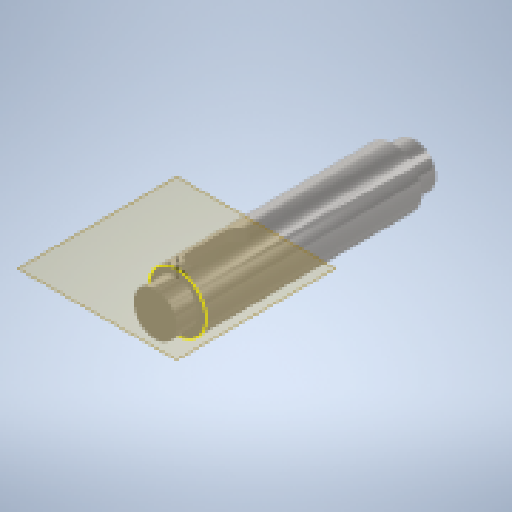
# Autodesk Inventor part: 入力軸
Saved by Autodesk Inventor 2024 (Build 280153000, 153)
## iProperties
Created: 2023-05-29
Part Number: 入力軸
Material: 鋼、炭素鋼
Document SubType Name: Modeling
Designer: yuta2
Density: 7.85 g/cm^3
Appearance: 半つや出し
Mass: 16.8186 g
Surface Area: 12.4913 cm^2
Volume: 2.1425 cm^3
Author: yuta2
Autodesk Inventor part; units mm, degrees
ref_plane "YZ Plane" through (0, 0, 0) normal (1, 0, 0) x (0, 1, 0)
ref_plane "XZ Plane" through (0, 0, 0) normal (0, 1, 0) x (-1, 0, 0)
ref_plane "XY Plane" through (0, 0, 0) normal (0, 0, 1) x (1, 0, 0)
sketch "スケッチ1" plane through (0, 0, 0) normal (1, 0, 0) x (0, 1, 0)
  line L0 (0, 0) -> (3, 0)
  line L1 (3, 0) -> (3, 3)
  line L2 (3, 3) -> (0, 3)
  line L3 (0, 3) -> (0, 0)
  line L4 (0, 0) -> (4, 0)
  line L5 (4, 0) -> (4, -37)
  line L6 (4, -37) -> (0, -37)
  line L7 (0, -37) -> (0, 0)
  line L8 (0, -37) -> (3, -37)
  line L9 (3, -37) -> (3, -40)
  line L10 (3, -40) -> (0, -40)
  line L11 (0, -40) -> (0, -37)
  dimension "d0" = 3
  dimension "d1" = 3
  dimension "d2" = 4
  dimension "d3" = 37
  dimension "d4" = 3
  dimension "d5" = 3
  constraints: 24 end point, 6 parallel, 3 horizontal, 3 perpendicular
  measures "d0" distance of L2.end L1.end
  measures "d1" distance of L1.end L0.end
  measures "d2" distance of L5.end L6.end
  measures "d3" distance of L4.end L5.end
  measures "d4" distance of L9.end L10.end
  measures "d5" distance of L8.end L9.end
revolve "回転1" add sketch "スケッチ1" angle 360 about axis through (0, 0, -37) along (0, 0, 1)
sketch "スケッチ2" plane through (0, 0, 0) normal (0, 0, 1) x (1, 0, 0)
  circle A0 centre (0, 0) radius 4 projected
  point P0 (0, 4)
  constraints: 2 vertical alignment, 1 other
ref_plane "作業平面1" through (0, 4, 0) normal (0, 1, 0) x (-1, 0, 0)
sketch "スケッチ3" plane through (0, 4, 0) normal (0, 1, 0) x (-1, 0, 0)
  line L0 (0, 0) -> (0, 3)
  line L1 (3, 3) -> (-3, 3) projected
  line L2 (1.5, -3) -> (-1.5, -3)
  line L3 (-1.5, -3) -> (-1.5, -8)
  line L4 (-1.5, -8) -> (1.5, -8)
  line L5 (1.5, -8) -> (1.5, -3)
  line L6 (4, 0) -> (-4, 0) projected
  circle A0 centre (0, -3) radius 1.5
  circle A1 centre (0, -8) radius 1.5
  line L7 (-1.5, -27) -> (1.5, -27)
  line L8 (1.5, -27) -> (1.5, -17)
  line L9 (1.5, -17) -> (-1.5, -17)
  line L10 (-1.5, -17) -> (-1.5, -27)
  circle A2 centre (0, -27) radius 1.5
  circle A3 centre (0, -17) radius 1.5
  dimension "d7" = 3
  dimension "d8" = 5
  dimension "d9" = 3
  dimension "d12" = 3
  dimension "d13" = 9
  dimension "d14" = 10
  constraints: 18 end point, 5 midpoint, 4 parallel, 2 horizontal, 2 perpendicular, 14 other
  measures "d7" distance between parallel lines of L6 L2
  measures "d8" distance of L2.end L3.end
  measures "d9" distance between parallel lines of L3 L5
  measures "d12" distance between parallel lines of L8 L10
  measures "d13" distance between parallel lines of L4 L9
  measures "d14" distance between parallel lines of L9 L7
extrude "押し出し1" cut sketch "スケッチ3" against normal blind 1.8
